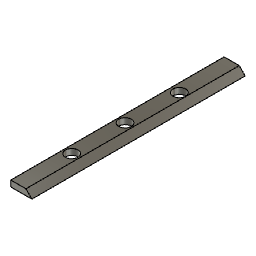
Dove_Tail_For_Main_Plate (Autodesk Fusion 360 design; units mm, degrees)
Autodesk Fusion 360 part; units mm, degrees
sketch "Sketch1" plane through (0, 0, 0) normal (0, 1, 0) x (1, 0, 0)
  line L0 (0, 0) -> (5.5118, 0)
  line L1 (0, 0) -> (0, -1.5748)
  line L2 (0, -1.5748) -> (3.9624, -1.5748)
  line L3 (3.9624, -1.5748) -> (5.5118, 0)
  dimension "d1" = 5.5118
  dimension "d2" = 1.5748
  constraint coincident L0.start L1.start
  constraint horizontal L0
  constraint perpendicular L0 L1
  constraint perpendicular L1 L2
  measures "d1" distance of L0.start L0.end
  measures "d2" distance of L0.start L1.end
extrude "Extrude1" add sketch "Sketch1" along normal blind 55.88
sketch "Sketch2" plane through (0, 0, 1.5748) normal (0, 0, 1) x (-1, 0, 0)
  line L0 (0, 0) -> (-3.9624, 0)
  line L1 (-3.9624, 0) -> (-3.9624, -55.88)
  line L2 (-3.9624, -55.88) -> (0, -55.88)
  line L3 (0, -55.88) -> (0, 0)
  line L4 (0, -55.88) -> (-3.9624, -55.88)
  line L5 (-3.9624, -55.88) -> (-3.9624, 0)
  line L6 (-3.9624, 0) -> (0, 0)
  line L7 (0, 0) -> (0, -55.88)
  line L8 (0, -27.94) -> (-3.9624, -27.94) construction
  circle A0 centre (-1.9812, -27.94) radius 1.6637
  line L9 (-1.9812, -27.94) -> (-1.9812, 0) construction
  circle A1 centre (-1.9812, -13.97) radius 1.6637
  circle A2 centre (-2.2352, -41.91) radius 1.6637
  dimension "d11" = 3.3274
  dimension "d12" = 3.3274
  dimension "d13" = 3.3274
  constraint horizontal L4
  constraint vertical L5
  constraint horizontal L6
  constraint vertical L7
  constraint coincident L0.end L1.start
  constraint coincident L2.end L3.start
  constraint midpoint L3 L8.start
  constraint midpoint L1 L8.end
  constraint midpoint L0 L9.end
  constraint midpoint L8 A0.centre
  constraint coincident A0.centre L9.start
  constraint midpoint L9 A1.centre
  measures "d11" diameter of A0
  measures "d12" diameter of A1
  measures "d13" diameter of A2
extrude "Extrude2" cut sketch "Sketch2" against normal blind 7.62 contours A0 | A1 | A2
